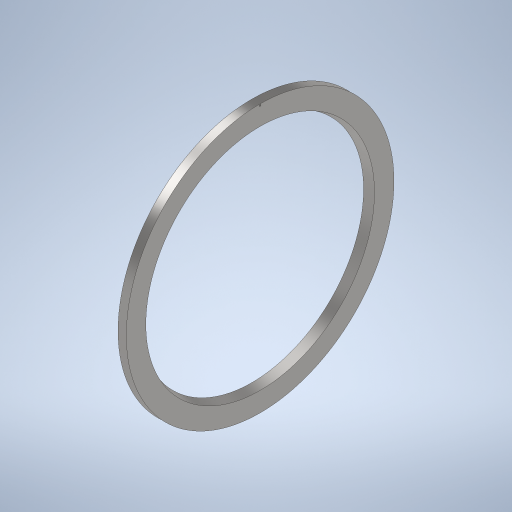
# Autodesk Inventor part: back bracket
Saved by Autodesk Inventor 2023 (Build 270158000, 158)
## iProperties
Created: 2022-07-21
Part Number: back bracket
Material: Stainless Steel
Document SubType Name: Modeling
Designer: station
Density: 8 g/cm^3
Appearance: Semi-Polished
Mass: 74.2938 g
Surface Area: 78.4029 cm^2
Volume: 9.28672 cm^3
Author: station
Autodesk Inventor part; units mm, degrees
ref_plane "YZ Plane" through (0, 0, 0) normal (1, 0, 0) x (0, 1, 0)
ref_plane "XZ Plane" through (0, 0, 0) normal (0, 1, 0) x (-1, 0, 0)
ref_plane "XY Plane" through (0, 0, 0) normal (0, 0, 1) x (1, 0, 0)
sketch "Sketch1" plane through (0, 0, 0) normal (0, 0, 1) x (1, 0, 0)
  arc A0 (180.1312, 23.4516) -> (181.5833, 23.6751) centre (180.1312, 28.2803) ccw
  arc A1 (180.1312, 23.4516) -> (181.5842, 23.6753) centre (180.1312, 28.2803) ccw
  arc A2 (167.724, 26.7761) -> (180.1312, 23.4516) centre (180.1312, 48.266) ccw
  arc A3 (166.724, 25.044) -> (180.1312, 21.4516) centre (180.1312, 48.266) ccw
  line L0 (125.6541, 47.7887) -> (168.987, 22.7705)
  line L1 (124.6541, 46.0566) -> (167.987, 21.0384)
  arc A4 (180.1312, 21.4516) -> (182.1847, 21.7676) centre (180.1312, 28.2803) ccw
  arc A5 (124.6541, 46.0566) -> (31.2848, 71.0749) centre (31.2848, -115.6637) ccw
  arc A6 (125.6541, 47.7887) -> (31.2848, 73.0749) centre (31.2848, -115.6637) ccw
  line L2 (1.263, 71.0749) -> (31.2848, 71.0749)
  line L3 (1.263, 73.0749) -> (31.2848, 73.0749)
  line L4 (236.5136, 40.9945) -> (181.5833, 23.6751)
  line L5 (182.1847, 21.7676) -> (237.115, 39.0871)
  line L6 (1.263, -0.4301) -> (320.4324, -0.4301)
  line L7 (236.5136, 40.9945) -> (237.115, 39.0871)
  line L8 (1.263, 84.1749) -> (31.2848, 84.1749)
  line L9 (167.987, 21.0384) -> (167.987, -8.65)
  line L10 (31.2848, 84.1749) -> (166.987, 84.1749)
  line L11 (233.5136, 47.8077) -> (145.7323, 20.1304)
  line L12 (234.2883, 48.052) -> (238.3779, 48.052)
  line L13 (234.2883, 48.052) -> (168.987, 48.052)
  line L14 (168.987, 86.1749) -> (31.2848, 86.1749)
  line L15 (31.2848, 86.1749) -> (1.263, 86.1749)
  line L16 (234.2883, 50.052) -> (170.987, 50.052)
  line L17 (169.987, 21.0384) -> (169.987, 27.7779)
  line L18 (169.987, 51.052) -> (169.987, 85.1749)
  line L19 (167.987, 21.0384) -> (167.987, 27.1473)
  line L20 (167.987, 49.052) -> (167.987, 83.1749)
  arc A7 (167.987, 83.1749) -> (166.987, 84.1749) centre (166.987, 83.1749) ccw
  arc A8 (169.987, 85.1749) -> (168.987, 86.1749) centre (168.987, 85.1749) ccw
  arc A9 (169.987, 51.052) -> (170.987, 50.052) centre (170.987, 51.052) ccw
  arc A10 (167.987, 49.052) -> (168.987, 48.052) centre (168.987, 49.052) ccw
  line L21 (1.263, 84.1749) -> (1.263, 86.1749)
  line L22 (238.3779, 48.052) -> (238.3779, 50.052)
  line L23 (234.2883, 50.052) -> (238.3779, 50.052)
  line L24 (236.5136, 40.9945) -> (236.5136, 48.052)
  line L25 (236.5136, 48.052) -> (233.5136, 48.052)
  line L26 (233.5136, 48.052) -> (233.5136, 40.0486)
  line L27 (233.5136, 48.052) -> (234.2883, 48.052)
  line L28 (233.5136, 48.052) -> (233.5136, 47.8077)
  dimension "d40" = 30.0219
  dimension "d41" = 186.7386
  dimension "d42" = 0
  dimension "d43" = 0
  dimension "d44" = 71.505
  dimension "d45" = 2
  dimension "d46" = 2
  dimension "d47" = 2
  dimension "d48" = 2
  dimension "d49" = 2
  dimension "d50" = 17.5
  dimension "d51" = 54.9303
  dimension "d52" = 2
  dimension "d53" = 11.1
  dimension "d54" = 7.4
  dimension "d55" = 17.5
  dimension "d56" = 2
  dimension "d57" = 2
  dimension "d58" = 1
  dimension "d59" = 1
  dimension "d60" = 1
  dimension "d61" = 1
  dimension "d62" = 3
  constraints: 58 end point, 22 point on circle, 11 centre point, 9 tangent, 6 point on line, 4 horizontal, 4 parallel, 4 vertical, 3 perpendicular, 1 collinear, 2 other
  measures "d40" distance of L2.start L2.end
  measures "d41" radius of A5
  measures "d42" distance of A5.end L2.end
  measures "d43" distance of L1.start A5.start
  measures "d44" distance between parallel lines of L6 L2
  measures "d45" distance between parallel lines of L2 L3
  measures "d46" radial gap between concentric circles of A5 A6
  measures "d47" distance between parallel lines of L1 L0
  measures "d48" radial gap between concentric circles of A3 A2
  measures "d49" radial gap between concentric circles of A4 A1
  measures "d50" angle of L6 L5
  measures "d51" horizontal distance of L5.start L5.end
  measures "d52" distance between parallel lines of L5 L4
  measures "d53" distance between parallel lines of L3 L8
  measures "d54" distance of L13.start L4.start
  measures "d55" angle of L6 L11
  measures "d56" distance between parallel lines of L10 L14
  measures "d57" distance between parallel lines of L13 L16
  measures "d58" radius of A7
  measures "d59" radius of A8
  measures "d60" radius of A9
  measures "d61" radius of A10
  measures "d62" distance of L24.end L25.end
revolve "Revolution1" add sketch "Sketch1" angle 360 about axis through (1.263, -0.4301, 0) along (1, 0, 0) contours L26 L13 L12 L24 L4
sketch "Sketch2" plane through (236.5136, -0.4301, 0) normal (1, 0, 0) x (0, 0, -1)
  circle A0 centre (0, 0) radius 41.4246 projected
  line L0 (0, 41.4246) -> (0, 46.1871)
  circle A1 centre (0, 46.1871) radius 4.7625
  point P0 (0, 0.4301)
  dimension "d63" = 4.7625
  dimension "d64" = 9.525
  constraints: 2 end point, 1 centre point, 1 coincident, 1 vertical, 1 vertical alignment, 1 other
  measures "d63" distance of L0.start L0.end
  measures "d64" diameter of A1
sketch "Sketch5" plane through (236.5136, -0.4301, 0) normal (1, 0, 0) x (0, 0, -1)
  circle A0 centre (0, 42.1815) radius 4.7625 projected
  circle A1 centre (0, 0) radius 48.4822 projected
  line L0 (0, 48.4822) -> (0, 47.9822)
  line L1 (0.25, 47.7322) -> (-0.25, 47.7322)
  line L2 (-0.25, 47.7322) -> (-0.25, 48.2322)
  line L3 (-0.25, 48.2322) -> (0.25, 48.2322)
  line L4 (0.25, 48.2322) -> (0.25, 47.7322)
  line L5 (0.25, 47.7322) -> (-0.25, 48.2322) construction
  line L6 (-0.25, 47.7322) -> (0.25, 48.2322) construction
  point P0 (0, 0.4301)
  point P1 (0, 41.4246)
  dimension "d72" = 0.5
  dimension "d76" = 0.5
  dimension "d77" = 0.5
  constraints: 14 end point, 2 midpoint, 2 parallel, 2 vertical alignment, 1 horizontal, 1 perpendicular, 1 vertical, 1 other
  measures "d72" distance of L0.start L0.end
  measures "d76" distance of L2.end L3.end
  measures "d77" distance of L1.end L2.end
extrude "Extrusion1" cut sketch "Sketch5" against normal blind 3.5 contours L3 L4 L1 L2
body "Solid1"
